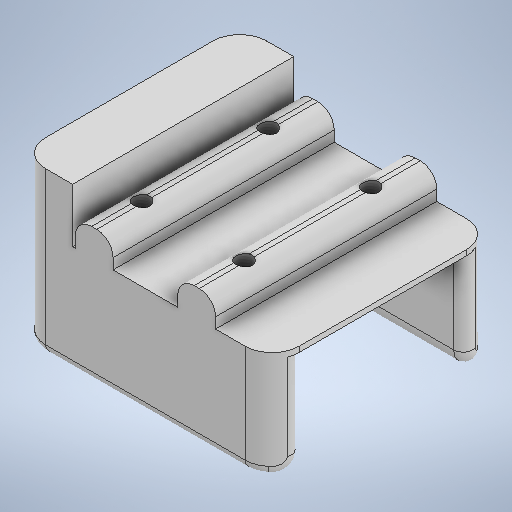
# Autodesk Inventor part: CaseInterno2.0
Saved by Autodesk Inventor 2025.2 (Build 292293000, 293)
## iProperties
Created: 2025-04-16
Part Number: CaseInterno2.0
Material: Genérico
Document SubType Name: Modeling
Designer: miche
Density: 1 g/cm^3
Appearance: Padrão
Author: miche
Autodesk Inventor part; units mm, degrees
ref_plane "YZ Plane" through (0, 0, 0) normal (1, 0, 0) x (0, 1, 0)
ref_plane "XZ Plane" through (0, 0, 0) normal (0, 1, 0) x (-1, 0, 0)
ref_plane "XY Plane" through (0, 0, 0) normal (0, 0, 1) x (1, 0, 0)
sketch "Esboço1" plane through (0, 0, 0) normal (0, 1, 0) x (-1, 0, 0)
  line L0 (0, 0) -> (-51, 0)
  line L1 (-51, 0) -> (-51, -45)
  line L2 (-51, -45) -> (0, -45)
  line L3 (0, -45) -> (0, 0)
  line L4 (0, -45) -> (-2, -45)
  line L5 (-2, -45) -> (-2, -43)
  line L6 (-2, -43) -> (0, -43)
  line L7 (0, -43) -> (0, -45)
  line L8 (-51, 0) -> (-49, 0)
  line L9 (-49, 0) -> (-49, -2)
  line L10 (-49, -2) -> (-51, -2)
  line L11 (-51, -2) -> (-51, 0)
  line L12 (-7, -43) -> (-44, -43)
  line L13 (-49, -38) -> (-49, -7)
  line L14 (-44, -2) -> (-7, -2)
  line L15 (-2, -7) -> (-2, -38)
  arc A0 (-7, -43) -> (-2, -38) centre (-7, -38) ccw
  arc A1 (-49, -38) -> (-44, -43) centre (-44, -38) ccw
  arc A2 (-44, -2) -> (-49, -7) centre (-44, -7) ccw
  arc A3 (-2, -7) -> (-7, -2) centre (-7, -7) ccw
  line L16 (-51, -45) -> (-35, -45)
  line L17 (-35, -45) -> (-16, -45)
  line L18 (-16, -45) -> (-16, -34.25)
  line L19 (-16, -34.25) -> (-35, -34.25)
  line L20 (-35, -34.25) -> (-35, -45)
  line L21 (-51, 0) -> (-35, 0)
  line L22 (-35, 0) -> (-16, 0)
  line L23 (-16, 0) -> (-16, -10.75)
  line L24 (-16, -10.75) -> (-35, -10.75)
  line L25 (-35, -10.75) -> (-35, 0)
  circle A4 centre (-35, -34.25) radius 1.5
  circle A5 centre (-16, -34.25) radius 1.5
  circle A6 centre (-35, -10.75) radius 1.5
  circle A7 centre (-16, -10.75) radius 1.5
  dimension "d0" = 51
  dimension "d1" = 45
  dimension "d2" = 5
  dimension "d5" = 16
  dimension "d6" = 19
  dimension "d7" = 10.75
  dimension "d8" = 16
  dimension "d9" = 10.75
  dimension "d10" = 3
  dimension "d11" = 3
  dimension "d12" = 3
  dimension "d13" = 3
  constraints: 52 end point, 12 parallel, 8 centre point, 8 point on circle, 8 tangent, 6 horizontal, 6 perpendicular, 6 point on line, 4 coincident, 3 equal radius
  measures "d0" distance of L2.end L1.end
  measures "d1" distance of L1.end L0.end
  measures "d2" radius of A0
  measures "d5" distance of L1.end L16.end
  measures "d6" distance of L19.end L18.end
  measures "d7" distance of L18.end L17.end
  measures "d8" distance of L0.end L21.end
  measures "d9" distance of L22.end L23.end
  measures "d10" diameter of A4
  measures "d11" diameter of A5
  measures "d12" diameter of A6
  measures "d13" diameter of A7
extrude "Extrusão1" add sketch "Esboço1" along normal blind 1 contours L23 A7 L24 A6 L25 L14 | L14 A3 L15 A0 L12 L18 A5 L19 A4 L20 A1 L13 A2 L25 A6 L24 A7 L23 | A7 L24 L23 | L23 L24 A7 | A6 L24 L25 | L25 L24 A6 | L12 L20 A4 L19 A5 L18 | A5 L19 L18 | L18 L19 A5 | A4 L19 L20 | L20 L19 A4
extrude "Extrusão2" cut sketch "Esboço1" along normal blind 10 contours A7 L24 L23 | L23 L24 A7 | A6 L24 L25 | L25 L24 A6 | A5 L19 L18 | L18 L19 A5 | A4 L19 L20 | L20 L19 A4
sketch "Esboço3" plane through (0, 1, 0) normal (0, 1, 0) x (1, 0, 0)
  circle A0 centre (35, 10.75) radius 1.5 projected
  line L0 (35, 10.75) -> (38.5, 10.75)
  line L1 (35, 10.75) -> (31.5, 10.75)
  line L2 (16, 10.75) -> (12.5, 10.75)
  line L3 (16, 10.75) -> (19.5, 10.75)
  line L4 (7, 2) -> (44, 2) projected
  line L5 (38.5, 2) -> (31.5, 2)
  line L6 (31.5, 2) -> (31.5, 43)
  line L7 (31.5, 43) -> (38.5, 43)
  line L8 (38.5, 43) -> (38.5, 2)
  line L9 (19.5, 2) -> (12.5, 2)
  line L10 (12.5, 2) -> (12.5, 43)
  line L11 (12.5, 43) -> (19.5, 43)
  line L12 (19.5, 43) -> (19.5, 2)
  circle A1 centre (35, 34.25) radius 1.5 projected
  circle A2 centre (35, 34.25) radius 1.5
  circle A3 centre (16, 34.25) radius 1.5
  circle A4 centre (16, 10.75) radius 1.5 projected
  circle A5 centre (16, 10.75) radius 1.5
  point P0 (0, 0)
  dimension "d16" = 3.5
  dimension "d17" = 3.5
  dimension "d18" = 3.5
  dimension "d19" = 3.5
  constraints: 24 end point, 6 horizontal, 4 parallel, 3 centre point, 3 point on line, 2 coincident, 2 perpendicular
  measures "d16" distance of L0.start L0.end
  measures "d17" distance of L0.start L1.end
  measures "d18" distance of L2.start L2.end
  measures "d19" distance of L2.start L3.end
extrude "Extrusão3" add sketch "Esboço3" along normal blind 5 contours L0 L8 L4 L6 L1 A0 | A0 L1 L6 L7 L8 L0 | A4 L3 L12 L4 L10 L2 | L2 L10 L11 L12 L3 A4
fillet "Arredondamento da face1" radius 3.03 1 edges at (12.5, 6, -22.5)
fillet "Arredondamento da face2" radius 3.03 1 edges at (19.5, 6, -22.5)
fillet "Arredondamento da face3" radius 3.03 1 edges at (31.5, 6, -22.5)
fillet "Arredondamento da face4" radius 3.03 1 edges at (38.5, 6, -22.5)
sketch "Esboço4" plane through (0, 0, 0) normal (0, -1, 0) x (1, 0, 0)
  line L0 (51, 0) -> (0, 0)
  line L1 (0, 0) -> (0, -7.5)
  line L2 (0, -7.5) -> (51, -7.5)
  line L3 (51, -7.5) -> (51, 0)
  line L4 (51, -45.199897) -> (0, -45.199897)
  line L5 (0, -45.199897) -> (0, -37.699897)
  line L6 (0, -37.699897) -> (51, -37.699897)
  line L7 (51, -37.699897) -> (51, -45.199897)
  arc A0 (49, -7) -> (44, -2) centre (44, -7) ccw
  arc A1 (49, -7) -> (44, -2) centre (44, -7) ccw
  arc A2 (44, -43) -> (49, -38) centre (44, -38) ccw
  arc A3 (44, -43) -> (49, -38) centre (44, -38) ccw
  arc A4 (2, -38) -> (7, -43) centre (7, -38) ccw
  arc A5 (2, -38) -> (7, -43) centre (7, -38) ccw
  arc A6 (7, -2) -> (2, -7) centre (7, -7) ccw
  arc A7 (7, -2) -> (2, -7) centre (7, -7) ccw
  line L8 (44, -2) -> (7, -2)
  line L9 (44, -43) -> (7, -43)
  line L10 (44, -43) -> (38.5, -43)
  line L11 (49, -7) -> (49, -38)
  line L12 (2, -38) -> (2, -7)
  line L13 (49, -7) -> (2, -7)
  line L14 (2, -7) -> (2, -38)
  line L15 (2, -38) -> (49, -38)
  line L16 (49, -38) -> (49, -7)
  point P0 (49, -37.699897)
  point P1 (2, -37.699897)
  point P2 (2, -7.5)
  point P3 (49, -7.5)
  dimension "d26" = 7.5
  dimension "d27" = 7.5
  constraints: 28 end point, 8 point on circle, 6 parallel, 4 centre point, 3 horizontal, 3 perpendicular, 2 point on line, 1 collinear
  measures "d26" distance of L1.end L0.end
  measures "d27" distance of L4.end L5.end
extrude "Extrusão4" add sketch "Esboço4" along normal blind 19 contours L2 L12 L13 L11 | L13 A6 L8 A0 | L11 L15 L12 L6 | A2 L9 A4 L15
fillet "Arredondamento da face5" radius 3.03 1 edges at (25.5, -19, -7.5)
fillet "Arredondamento da face6" radius 3.03 1 edges at (25.5, -19, -37.6999)
fillet "Arredondamento da face7" radius 1.71 1 edges at (25.5, -19, -2)
fillet "Arredondamento da face8" radius 1.71 1 edges at (25.5, -19, -43)
sketch "Esboço5" plane through (0, 1, 0) normal (0, 1, 0) x (1, 0, 0)
  line L0 (12.5, 2) -> (12.5, 43)
  line L1 (12.5, 2) -> (12, 2)
  line L2 (12, 2) -> (12, 43)
  line L3 (12, 43) -> (12.5, 43)
  line L4 (12.5, 43) -> (12.5, 2)
  line L5 (7, 2) -> (12.5, 2)
  line L6 (12, 2) -> (7, 2)
  line L7 (12.5, 43) -> (7, 43)
  line L8 (12, 43) -> (7, 43)
  arc A0 (2, 7) -> (2.350438, 5.161094) centre (7, 7) ccw
  line L9 (2, 7) -> (2, 38)
  line L10 (2, 7) -> (2, 38)
  arc A1 (7, 43) -> (2, 38) centre (7, 38) ccw
  arc A2 (3.803738, 3.155015) -> (7, 2) centre (7, 7) ccw
  arc A3 (2, 7) -> (7, 2) centre (7, 7) ccw
  point P0 (0, 0)
  point P1 (2.350438, 5.161094)
  constraints: 14 end point, 5 point on circle, 2 centre point, 2 horizontal, 2 parallel, 1 collinear, 1 perpendicular, 1 tangent, 1 vertical
extrude "Extrusão5" add sketch "Esboço5" along normal blind 10 contours L5 A2 A3 A0 L9 A1 L7 L2
thread "Rosca1" size "M3x0.5" class "6H" standard "ANSI Metric M Profile" length 10
thread "Rosca2" size "M3x0.5" class "6H" standard "ANSI Metric M Profile" length 10
thread "Rosca3" size "M3x0.5" class "6H" standard "ANSI Metric M Profile" length 10
thread "Rosca4" size "M3x0.5" class "6H" standard "ANSI Metric M Profile" length 10
fillet "Arredondamento da face9" radius 1.71 1 edges at (2, 0, -22.5)
